Autodesk Inventor part; units mm, degrees
(part 3 of 3)
chamfer "面取り1" distance 0.1 angle 45 1544 edges at (166.6875, 1.524, 45.7073) (173.6108, 1.524, 45.7817) (173.6852, 1.524, 52.705) (173.6108, 1.524, 59.6283) (166.6875, 1.524, 59.7027) (159.7642, 1.524, 59.6283) (159.6898, 1.524, 52.705) (159.7642, 1.524, 45.7817) (166.6875, 0, 45.7073) (173.6108, 0, 45.7817) (173.6852, 0, 52.705) (173.6108, 0, 59.6283) (166.6875, 0, 59.7027) (159.7642, 0, 59.6283) (159.6898, 0, 52.705) (159.7642, 0, 45.7817) (147.6375, 1.524, 45.7073) (154.5608, 1.524, 45.7817) (154.6352, 1.524, 52.705) (154.5608, 1.524, 59.6283) (147.6375, 1.524, 59.7027) (140.7142, 1.524, 59.6283) (140.6398, 1.524, 52.705) (140.7142, 1.524, 45.7817) (147.6375, 0, 45.7073) (154.5608, 0, 45.7817) (154.6352, 0, 52.705) (154.5608, 0, 59.6283) (147.6375, 0, 59.7027) (140.7142, 0, 59.6283) (140.6398, 0, 52.705) (140.7142, 0, 45.7817) (128.5875, 0, 45.7073) (135.5108, 0, 45.7817) (135.5852, 0, 52.705) (135.5108, 0, 59.6283) (128.5875, 0, 59.7027) (121.6642, 0, 59.6283) (121.5898, 0, 52.705) (121.6642, 0, 45.7817) (128.5875, 1.524, 45.7073) (135.5108, 1.524, 45.7817) (135.5852, 1.524, 52.705) (135.5108, 1.524, 59.6283) (128.5875, 1.524, 59.7027) (121.6642, 1.524, 59.6283) (121.5898, 1.524, 52.705) (121.6642, 1.524, 45.7817) (147.6375, 1.524, 26.6573) (154.5608, 1.524, 26.7317) (154.6352, 1.524, 33.655) (154.5608, 1.524, 40.5783) (147.6375, 1.524, 40.6527) (140.7142, 1.524, 40.5783) (140.6398, 1.524, 33.655) (140.7142, 1.524, 26.7317) (147.6375, 0, 26.6573) (154.5608, 0, 26.7317) (154.6352, 0, 33.655) (154.5608, 0, 40.5783) (147.6375, 0, 40.6527) (140.7142, 0, 40.5783) (140.6398, 0, 33.655) (140.7142, 0, 26.7317) (97.63, 1.524, 45.7073) (104.5533, 1.524, 45.7817) (104.6277, 1.524, 52.705) (104.5533, 1.524, 59.6283) (97.63, 1.524, 59.7027) (90.7067, 1.524, 59.6283) (90.6323, 1.524, 52.705) (90.7067, 1.524, 45.7817) (97.63, 0, 45.7073) (104.5533, 0, 45.7817) (104.6277, 0, 52.705) (104.5533, 0, 59.6283) (97.63, 0, 59.7027) (90.7067, 0, 59.6283) (90.6323, 0, 52.705) (90.7067, 0, 45.7817) (73.8175, 1.524, 45.7073) (80.7408, 1.524, 45.7817) (80.8152, 1.524, 52.705) (80.7408, 1.524, 59.6283) (73.8175, 1.524, 59.7027) (66.8942, 1.524, 59.6283) (66.8198, 1.524, 52.705) (66.8942, 1.524, 45.7817) (73.8175, 0, 45.7073) (80.7408, 0, 45.7817) (80.8152, 0, 52.705) (80.7408, 0, 59.6283) (73.8175, 0, 59.7027) (66.8942, 0, 59.6283) (66.8198, 0, 52.705) (66.8942, 0, 45.7817) (78.4531, 0, 28.2829) (81.8787, 0, 28.3573) (81.9531, 0, 33.9979) (81.8787, 0, 39.6385) (78.4531, 0, 39.7129) (75.0275, 0, 39.6385) (74.9531, 0, 33.9979) (75.0275, 0, 28.3573) (78.4531, 1.524, 28.2829) (81.8787, 1.524, 28.3573) (81.9531, 1.524, 33.9979) (81.8787, 1.524, 39.6385) (78.4531, 1.524, 39.7129) (75.0275, 1.524, 39.6385) (74.9531, 1.524, 33.9979) (75.0275, 1.524, 28.3573) (90.4875, 1.524, 26.6573) (97.4108, 1.524, 26.7317) (97.4852, 1.524, 33.655) (97.4108, 1.524, 40.5783) (90.4875, 1.524, 40.6527) (83.5642, 1.524, 40.5783) (83.4898, 1.524, 33.655) (83.5642, 1.524, 26.7317) (90.4875, 0, 26.6573) (97.4108, 0, 26.7317) (97.4852, 0, 33.655) (97.4108, 0, 40.5783) (90.4875, 0, 40.6527) (83.5642, 0, 40.5783) (83.4898, 0, 33.655) (83.5642, 0, 26.7317) (102.5219, 0, 28.2829) (105.9475, 0, 28.3573) (106.0219, 0, 33.9979) (105.9475, 0, 39.6385) (102.5219, 0, 39.7129) (99.0963, 0, 39.6385) (99.0219, 0, 33.9979) (99.0963, 0, 28.3573) (102.5219, 1.524, 28.2829) (105.9475, 1.524, 28.3573) (106.0219, 1.524, 33.9979) (105.9475, 1.524, 39.6385) (102.5219, 1.524, 39.7129) (99.0963, 1.524, 39.6385) (99.0219, 1.524, 33.9979) (99.0963, 1.524, 28.3573) (97.9729, 0, 13.6144) (103.6135, 0, 13.6888) (103.6879, 0, 17.018) (103.6135, 0, 20.3472) (97.9729, 0, 20.4216) (92.3323, 0, 20.3472) (92.2579, 0, 17.018) (92.3323, 0, 13.6888) (97.9729, 1.524, 13.6144) (103.6135, 1.524, 13.6888) (103.6879, 1.524, 17.018) (103.6135, 1.524, 20.3472) (97.9729, 1.524, 20.4216) (92.3323, 1.524, 20.3472) (92.2579, 1.524, 17.018) (92.3323, 1.524, 13.6888) (97.63, 0, -1.9177) (104.5533, 0, -1.8433) (104.6277, 0, 5.08) (104.5533, 0, 12.0033) (97.63, 0, 12.0777) (90.7067, 0, 12.0033) (90.6323, 0, 5.08) (90.7067, 0, -1.8433) (97.63, 1.524, -1.9177) (104.5533, 1.524, -1.8433) (104.6277, 1.524, 5.08) (104.5533, 1.524, 12.0033) (97.63, 1.524, 12.0777) (90.7067, 1.524, 12.0033) (90.6323, 1.524, 5.08) (90.7067, 1.524, -1.8433) (97.9729, 0, -10.2616) (103.6135, 0, -10.1872) (103.6879, 0, -6.858) (103.6135, 0, -3.5288) (97.9729, 0, -3.4544) (92.3323, 0, -3.5288) (92.2579, 0, -6.858) (92.3323, 0, -10.1872) (97.9729, 1.524, -10.2616) (103.6135, 1.524, -10.1872) (103.6879, 1.524, -6.858) (103.6135, 1.524, -3.5288) (97.9729, 1.524, -3.4544) (92.3323, 1.524, -3.5288) (92.2579, 1.524, -6.858) (92.3323, 1.524, -10.1872) (100.0125, 0, -30.4927) (106.9358, 0, -30.4183) (107.0102, 0, -23.495) (106.9358, 0, -16.5717) (100.0125, 0, -16.4973) (93.0892, 0, -16.5717) (93.0148, 0, -23.495) (93.0892, 0, -30.4183) (100.0125, 1.524, -30.4927) (106.9358, 1.524, -30.4183) (107.0102, 1.524, -23.495) (106.9358, 1.524, -16.5717) (100.0125, 1.524, -16.4973) (93.0892, 1.524, -16.5717) (93.0148, 1.524, -23.495) (93.0892, 1.524, -30.4183) (100.0125, 0, -59.0677) (106.9358, 0, -58.9933) (107.0102, 0, -52.07) (106.9358, 0, -45.1467) (100.0125, 0, -45.0723) (93.0892, 0, -45.1467) (93.0148, 0, -52.07) (93.0892, 0, -58.9933) (100.0125, 1.524, -59.0677) (106.9358, 1.524, -58.9933) (107.0102, 1.524, -52.07) (106.9358, 1.524, -45.1467) (100.0125, 1.524, -45.0723) (93.0892, 1.524, -45.1467) (93.0148, 1.524, -52.07) (93.0892, 1.524, -58.9933) (128.5875, 0, -30.4927) (135.5108, 0, -30.4183) (135.5852, 0, -23.495) (135.5108, 0, -16.5717) (128.5875, 0, -16.4973) (121.6642, 0, -16.5717) (121.5898, 0, -23.495) (121.6642, 0, -30.4183) (128.5875, 1.524, -30.4927) (135.5108, 1.524, -30.4183) (135.5852, 1.524, -23.495) (135.5108, 1.524, -16.5717) (128.5875, 1.524, -16.4973) (121.6642, 1.524, -16.5717) (121.5898, 1.524, -23.495) (121.6642, 1.524, -30.4183) (128.5875, 0, -11.4427) (135.5108, 0, -11.3683) (135.5852, 0, -4.445) (135.5108, 0, 2.4783) (128.5875, 0, 2.5527) (121.6642, 0, 2.4783) (121.5898, 0, -4.445) (121.6642, 0, -11.3683) (128.5875, 1.524, -11.4427) (135.5108, 1.524, -11.3683) (135.5852, 1.524, -4.445) (135.5108, 1.524, 2.4783) (128.5875, 1.524, 2.5527) (121.6642, 1.524, 2.4783) (121.5898, 1.524, -4.445) (121.6642, 1.524, -11.3683) (147.6375, 1.524, -11.4427) (154.5608, 1.524, -11.3683) (154.6352, 1.524, -4.445) (154.5608, 1.524, 2.4783) (147.6375, 1.524, 2.5527) (140.7142, 1.524, 2.4783) (140.6398, 1.524, -4.445) (140.7142, 1.524, -11.3683) (147.6375, 0, -11.4427) (154.5608, 0, -11.3683) (154.6352, 0, -4.445) (154.5608, 0, 2.4783) (147.6375, 0, 2.5527) (140.7142, 0, 2.4783) (140.6398, 0, -4.445) (140.7142, 0, -11.3683) (147.6375, 0, -30.4927) (154.5608, 0, -30.4183) (154.6352, 0, -23.495) (154.5608, 0, -16.5717) (147.6375, 0, -16.4973) (140.7142, 0, -16.5717) (140.6398, 0, -23.495) (140.7142, 0, -30.4183) (147.6375, 1.524, -30.4927) (154.5608, 1.524, -30.4183) (154.6352, 1.524, -23.495) (154.5608, 1.524, -16.5717) (147.6375, 1.524, -16.4973) (140.7142, 1.524, -16.5717) (140.6398, 1.524, -23.495) (140.7142, 1.524, -30.4183) (166.6875, 0, -11.4427) (173.6108, 0, -11.3683) (173.6852, 0, -4.445) (173.6108, 0, 2.4783) (166.6875, 0, 2.5527) (159.7642, 0, 2.4783) (159.6898, 0, -4.445) (159.7642, 0, -11.3683) (166.6875, 1.524, -11.4427) (173.6108, 1.524, -11.3683) (173.6852, 1.524, -4.445) (173.6108, 1.524, 2.4783) (166.6875, 1.524, 2.5527) (159.7642, 1.524, 2.4783) (159.6898, 1.524, -4.445) (159.7642, 1.524, -11.3683) (166.6875, 0, -30.4927) (173.6108, 0, -30.4183) (173.6852, 0, -23.495) (173.6108, 0, -16.5717) (166.6875, 0, -16.4973) (159.7642, 0, -16.5717) (159.6898, 0, -23.495) (159.7642, 0, -30.4183) (166.6875, 1.524, -30.4927) (173.6108, 1.524, -30.4183) (173.6852, 1.524, -23.495) (173.6108, 1.524, -16.5717) (166.6875, 1.524, -16.4973) (159.7642, 1.524, -16.5717) (159.6898, 1.524, -23.495) (159.7642, 1.524, -30.4183) (80.9625, 0, -59.0677) (87.8858, 0, -58.9933) (87.9602, 0, -52.07) (87.8858, 0, -45.1467) (80.9625, 0, -45.0723) (74.0392, 0, -45.1467) (73.9648, 0, -52.07) (74.0392, 0, -58.9933) (80.9625, 1.524, -59.0677) (87.8858, 1.524, -58.9933) (87.9602, 1.524, -52.07) (87.8858, 1.524, -45.1467) (80.9625, 1.524, -45.0723) (74.0392, 1.524, -45.1467) (73.9648, 1.524, -52.07) (74.0392, 1.524, -58.9933) (80.9625, 1.524, -30.4927) (87.8858, 1.524, -30.4183) (87.9602, 1.524, -23.495) (87.8858, 1.524, -16.5717) (80.9625, 1.524, -16.4973) (74.0392, 1.524, -16.5717) (73.9648, 1.524, -23.495) (74.0392, 1.524, -30.4183) (80.9625, 0, -30.4927) (87.8858, 0, -30.4183) (87.9602, 0, -23.495) (87.8858, 0, -16.5717) (80.9625, 0, -16.4973) (74.0392, 0, -16.5717) (73.9648, 0, -23.495) (74.0392, 0, -30.4183) (71.4375, 0, -11.4427) (78.3608, 0, -11.3683) (78.4352, 0, -4.445) (78.3608, 0, 2.4783) (71.4375, 0, 2.5527) (64.5142, 0, 2.4783) (64.4398, 0, -4.445) (64.5142, 0, -11.3683) (71.4375, 1.524, -11.4427) (78.3608, 1.524, -11.3683) (78.4352, 1.524, -4.445) (78.3608, 1.524, 2.4783) (71.4375, 1.524, 2.5527) (64.5142, 1.524, 2.4783) (64.4398, 1.524, -4.445) (64.5142, 1.524, -11.3683) (76.2, 0, 7.6073) (83.1233, 0, 7.6817) (83.1977, 0, 14.605) (83.1233, 0, 21.5283) (76.2, 0, 21.6027) (69.2767, 0, 21.5283) (69.2023, 0, 14.605) (69.2767, 0, 7.6817) (76.2, 1.524, 7.6073) (83.1233, 1.524, 7.6817) (83.1977, 1.524, 14.605) (83.1233, 1.524, 21.5283) (76.2, 1.524, 21.6027) (69.2767, 1.524, 21.5283) (69.2023, 1.524, 14.605) (69.2767, 1.524, 7.6817) (50.005, 0, 45.7073) (56.9283, 0, 45.7817) (57.0027, 0, 52.705) (56.9283, 0, 59.6283) (50.005, 0, 59.7027) (43.0817, 0, 59.6283) (43.0073, 0, 52.705) (43.0817, 0, 45.7817) (50.005, 1.524, 45.7073) (56.9283, 1.524, 45.7817) (57.0027, 1.524, 52.705) (56.9283, 1.524, 59.6283) (50.005, 1.524, 59.7027) (43.0817, 1.524, 59.6283) (43.0073, 1.524, 52.705) (43.0817, 1.524, 45.7817) (61.9125, 0, 26.6573) (68.8358, 0, 26.7317) (68.9102, 0, 33.655) (68.8358, 0, 40.5783) (61.9125, 0, 40.6527) (54.9892, 0, 40.5783) (54.9148, 0, 33.655) (54.9892, 0, 26.7317) (61.9125, 1.524, 26.6573) (68.8358, 1.524, 26.7317) (68.9102, 1.524, 33.655) (68.8358, 1.524, 40.5783) (61.9125, 1.524, 40.6527) (54.9892, 1.524, 40.5783) (54.9148, 1.524, 33.655) (54.9892, 1.524, 26.7317) (57.15, 0, 7.6073) (64.0733, 0, 7.6817) (64.1477, 0, 14.605) (64.0733, 0, 21.5283) (57.15, 0, 21.6027) (50.2267, 0, 21.5283) (50.1523, 0, 14.605) (50.2267, 0, 7.6817) (57.15, 1.524, 7.6073) (64.0733, 1.524, 7.6817) (64.1477, 1.524, 14.605) (64.0733, 1.524, 21.5283) (57.15, 1.524, 21.6027) (50.2267, 1.524, 21.5283) (50.1523, 1.524, 14.605) (50.2267, 1.524, 7.6817) (52.3875, 0, -11.4427) (59.3108, 0, -11.3683) (59.3852, 0, -4.445) (59.3108, 0, 2.4783) (52.3875, 0, 2.5527) (45.4642, 0, 2.4783) (45.3898, 0, -4.445) (45.4642, 0, -11.3683) (52.3875, 1.524, -11.4427) (59.3108, 1.524, -11.3683) (59.3852, 1.524, -4.445) (59.3108, 1.524, 2.4783) (52.3875, 1.524, 2.5527) (45.4642, 1.524, 2.4783) (45.3898, 1.524, -4.445) (45.4642, 1.524, -11.3683) (61.9125, 0, -30.4927) (68.8358, 0, -30.4183) (68.9102, 0, -23.495) (68.8358, 0, -16.5717) (61.9125, 0, -16.4973) (54.9892, 0, -16.5717) (54.9148, 0, -23.495) (54.9892, 0, -30.4183) (61.9125, 1.524, -30.4927) (68.8358, 1.524, -30.4183) (68.9102, 1.524, -23.495) (68.8358, 1.524, -16.5717) (61.9125, 1.524, -16.4973) (54.9892, 1.524, -16.5717) (54.9148, 1.524, -23.495) (54.9892, 1.524, -30.4183) (61.9125, 0, -59.0677) (68.8358, 0, -58.9933) (68.9102, 0, -52.07) (68.8358, 0, -45.1467) (61.9125, 0, -45.0723) (54.9892, 0, -45.1467) (54.9148, 0, -52.07) (54.9892, 0, -58.9933) (61.9125, 1.524, -59.0677) (68.8358, 1.524, -58.9933) (68.9102, 1.524, -52.07) (68.8358, 1.524, -45.1467) (61.9125, 1.524, -45.0723) (54.9892, 1.524, -45.1467) (54.9148, 1.524, -52.07) (54.9892, 1.524, -58.9933) (42.8625, 1.524, -59.0677) (49.7858, 1.524, -58.9933) (49.8602, 1.524, -52.07) (49.7858, 1.524, -45.1467) (42.8625, 1.524, -45.0723) (35.9392, 1.524, -45.1467) (35.8648, 1.524, -52.07) (35.9392, 1.524, -58.9933) (42.8625, 0, -59.0677) (49.7858, 0, -58.9933) (49.8602, 0, -52.07) (49.7858, 0, -45.1467) (42.8625, 0, -45.0723) (35.9392, 0, -45.1467) (35.8648, 0, -52.07) (35.9392, 0, -58.9933) (42.8625, 0, -30.4927) (49.7858, 0, -30.4183) (49.8602, 0, -23.495) (49.7858, 0, -16.5717) (42.8625, 0, -16.4973) (35.9392, 0, -16.5717) (35.8648, 0, -23.495) (35.9392, 0, -30.4183) (42.8625, 1.524, -30.4927) (49.7858, 1.524, -30.4183) (49.8602, 1.524, -23.495) (49.7858, 1.524, -16.5717) (42.8625, 1.524, -16.4973) (35.9392, 1.524, -16.5717) (35.8648, 1.524, -23.495) (35.9392, 1.524, -30.4183) (42.8625, 0, 26.6573) (49.7858, 0, 26.7317) (49.8602, 0, 33.655) (49.7858, 0, 40.5783) (42.8625, 0, 40.6527) (35.9392, 0, 40.5783) (35.8648, 0, 33.655) (35.9392, 0, 26.7317) (42.8625, 1.524, 26.6573) (49.7858, 1.524, 26.7317) (49.8602, 1.524, 33.655) (49.7858, 1.524, 40.5783) (42.8625, 1.524, 40.6527) (35.9392, 1.524, 40.5783) (35.8648, 1.524, 33.655) (35.9392, 1.524, 26.7317) (38.1, 0, 7.6073) (45.0233, 0, 7.6817) (45.0977, 0, 14.605) (45.0233, 0, 21.5283) (38.1, 0, 21.6027) (31.1767, 0, 21.5283) (31.1023, 0, 14.605) (31.1767, 0, 7.6817) (38.1, 1.524, 7.6073) (45.0233, 1.524, 7.6817) (45.0977, 1.524, 14.605) (45.0233, 1.524, 21.5283) (38.1, 1.524, 21.6027) (31.1767, 1.524, 21.5283) (31.1023, 1.524, 14.605) (31.1767, 1.524, 7.6817) (33.3375, 0, -11.4427) (40.2608, 0, -11.3683) (40.3352, 0, -4.445) (40.2608, 0, 2.4783) (33.3375, 0, 2.5527) (26.4142, 0, 2.4783) (26.3398, 0, -4.445) (26.4142, 0, -11.3683) (33.3375, 1.524, -11.4427) (40.2608, 1.524, -11.3683) (40.3352, 1.524, -4.445) (40.2608, 1.524, 2.4783) (33.3375, 1.524, 2.5527) (26.4142, 1.524, 2.4783) (26.3398, 1.524, -4.445) (26.4142, 1.524, -11.3683) (23.8125, 0, -30.4927) (30.7358, 0, -30.4183) (30.8102, 0, -23.495) (30.7358, 0, -16.5717) (23.8125, 0, -16.4973) (16.8892, 0, -16.5717) (16.8148, 0, -23.495) (16.8892, 0, -30.4183) (23.8125, 1.524, -30.4927) (30.7358, 1.524, -30.4183) (30.8102, 1.524, -23.495) (30.7358, 1.524, -16.5717) (23.8125, 1.524, -16.4973) (16.8892, 1.524, -16.5717) (16.8148, 1.524, -23.495) (16.8892, 1.524, -30.4183) (26.1925, 0, 45.7073) (33.1158, 0, 45.7817) (33.1902, 0, 52.705) (33.1158, 0, 59.6283) (26.1925, 0, 59.7027) (19.2692, 0, 59.6283) (19.1948, 0, 52.705) (19.2692, 0, 45.7817) (26.1925, 1.524, 45.7073) (33.1158, 1.524, 45.7817) (33.1902, 1.524, 52.705) (33.1158, 1.524, 59.6283) (26.1925, 1.524, 59.7027) (19.2692, 1.524, 59.6283) (19.1948, 1.524, 52.705) (19.2692, 1.524, 45.7817) (23.8125, 0, 26.6573) (30.7358, 0, 26.7317) (30.8102, 0, 33.655) (30.7358, 0, 40.5783) (23.8125, 0, 40.6527) (16.8892, 0, 40.5783) (16.8148, 0, 33.655) (16.8892, 0, 26.7317) (23.8125, 1.524, 26.6573) (30.7358, 1.524, 26.7317) (30.8102, 1.524, 33.655) (30.7358, 1.524, 40.5783) (23.8125, 1.524, 40.6527) (16.8892, 1.524, 40.5783) (16.8148, 1.524, 33.655) (16.8892, 1.524, 26.7317) (19.05, 0, 7.6073) (25.9733, 0, 7.6817) (26.0477, 0, 14.605) (25.9733, 0, 21.5283) (19.05, 0, 21.6027) (12.1267, 0, 21.5283) (12.0523, 0, 14.605) (12.1267, 0, 7.6817) (19.05, 1.524, 7.6073) (25.9733, 1.524, 7.6817) (26.0477, 1.524, 14.605) (25.9733, 1.524, 21.5283) (19.05, 1.524, 21.6027) (12.1267, 1.524, 21.5283) (12.0523, 1.524, 14.605) (12.1267, 1.524, 7.6817) (14.2875, 0, -11.4427) (21.2108, 0, -11.3683) (21.2852, 0, -4.445) (21.2108, 0, 2.4783) (14.2875, 0, 2.5527) (7.3642, 0, 2.4783) (7.2898, 0, -4.445) (7.3642, 0, -11.3683) (14.2875, 1.524, -11.4427) (21.2108, 1.524, -11.3683) (21.2852, 1.524, -4.445) (21.2108, 1.524, 2.4783) (14.2875, 1.524, 2.5527) (7.3642, 1.524, 2.4783) (7.2898, 1.524, -4.445) (7.3642, 1.524, -11.3683) (14.2875, 0, -59.0677) (21.2108, 0, -58.9933) (21.2852, 0, -52.07) (21.2108, 0, -45.1467) (14.2875, 0, -45.0723) (7.3642, 0, -45.1467) (7.2898, 0, -52.07) (7.3642, 0, -58.9933) (14.2875, 1.524, -59.0677) (21.2108, 1.524, -58.9933) (21.2852, 1.524, -52.07) (21.2108, 1.524, -45.1467) (14.2875, 1.524, -45.0723) (7.3642, 1.524, -45.1467) (7.2898, 1.524, -52.07) (7.3642, 1.524, -58.9933) (4.7625, 0, -30.4927) (11.6858, 0, -30.4183) (11.7602, 0, -23.495) (11.6858, 0, -16.5717) (4.7625, 0, -16.4973) (-2.1608, 0, -16.5717) (-2.2352, 0, -23.495) (-2.1608, 0, -30.4183) (4.7625, 1.524, -30.4927) (11.6858, 1.524, -30.4183) (11.7602, 1.524, -23.495) (11.6858, 1.524, -16.5717) (4.7625, 1.524, -16.4973) (-2.1608, 1.524, -16.5717) (-2.2352, 1.524, -23.495) (-2.1608, 1.524, -30.4183) (-4.7625, 0, -59.0677) (2.1608, 0, -58.9933) (2.2352, 0, -52.07) (2.1608, 0, -45.1467) (-4.7625, 0, -45.0723) (-11.6858, 0, -45.1467) (-11.7602, 0, -52.07) (-11.6858, 0, -58.9933) (-4.7625, 1.524, -59.0677) (2.1608, 1.524, -58.9933) (2.2352, 1.524, -52.07) (2.1608, 1.524, -45.1467) (-4.7625, 1.524, -45.0723) (-11.6858, 1.524, -45.1467) (-11.7602, 1.524, -52.07) (-11.6858, 1.524, -58.9933) (4.7625, 0, 26.6573) (11.6858, 0, 26.7317) (11.7602, 0, 33.655) (11.6858, 0, 40.5783) (4.7625, 0, 40.6527) (-2.1608, 0, 40.5783) (-2.2352, 0, 33.655) (-2.1608, 0, 26.7317) (4.7625, 1.524, 26.6573) (11.6858, 1.524, 26.7317) (11.7602, 1.524, 33.655) (11.6858, 1.524, 40.5783) (4.7625, 1.524, 40.6527) (-2.1608, 1.524, 40.5783) (-2.2352, 1.524, 33.655) (-2.1608, 1.524, 26.7317) (0, 0, 7.6073) (6.9233, 0, 7.6817) (6.9977, 0, 14.605) (6.9233, 0, 21.5283) (0, 0, 21.6027) (-6.9233, 0, 21.5283) (-6.9977, 0, 14.605) (-6.9233, 0, 7.6817) (0, 1.524, 7.6073) (6.9233, 1.524, 7.6817) (6.9977, 1.524, 14.605) (6.9233, 1.524, 21.5283) (0, 1.524, 21.6027) (-6.9233, 1.524, 21.5283) (-6.9977, 1.524, 14.605) (-6.9233, 1.524, 7.6817) (-4.7625, 0, -11.4427) (2.1608, 0, -11.3683) (2.2352, 0, -4.445) (2.1608, 0, 2.4783) (-4.7625, 0, 2.5527) (-11.6858, 0, 2.4783) (-11.7602, 0, -4.445) (-11.6858, 0, -11.3683) (-4.7625, 1.524, -11.4427) (2.1608, 1.524, -11.3683) (2.2352, 1.524, -4.445) (2.1608, 1.524, 2.4783) (-4.7625, 1.524, 2.5527) (-11.6858, 1.524, 2.4783) (-11.7602, 1.524, -4.445) (-11.6858, 1.524, -11.3683) (-14.2875, 0, -30.4927) (-7.3642, 0, -30.4183) (-7.2898, 0, -23.495) (-7.3642, 0, -16.5717) (-14.2875, 0, -16.4973) (-21.2108, 0, -16.5717) (-21.2852, 0, -23.495) (-21.2108, 0, -30.4183) (-14.2875, 1.524, -30.4927) (-7.3642, 1.524, -30.4183) (-7.2898, 1.524, -23.495) (-7.3642, 1.524, -16.5717) (-14.2875, 1.524, -16.4973) (-21.2108, 1.524, -16.5717) (-21.2852, 1.524, -23.495) (-21.2108, 1.524, -30.4183) (-7.9375, 0, 47.3329) (-4.5119, 0, 47.4073) (-4.4375, 0, 53.0479) (-4.5119, 0, 58.6885) (-7.9375, 0, 58.7629) (-11.3631, 0, 58.6885) (-11.4375, 0, 53.0479) (-11.3631, 0, 47.4073) (-7.9375, 1.524, 47.3329) (-4.5119, 1.524, 47.4073) (-4.4375, 1.524, 53.0479) (-4.5119, 1.524, 58.6885) (-7.9375, 1.524, 58.7629) (-11.3631, 1.524, 58.6885) (-11.4375, 1.524, 53.0479) (-11.3631, 1.524, 47.4073) (-14.2875, 0, 26.6573) (-7.3642, 0, 26.7317) (-7.2898, 0, 33.655) (-7.3642, 0, 40.5783) (-14.2875, 0, 40.6527) (-21.2108, 0, 40.5783) (-21.2852, 0, 33.655) (-21.2108, 0, 26.7317) (-14.2875, 1.524, 26.6573) (-7.3642, 1.524, 26.7317) (-7.2898, 1.524, 33.655) (-7.3642, 1.524, 40.5783) (-14.2875, 1.524, 40.6527) (-21.2108, 1.524, 40.5783) (-21.2852, 1.524, 33.655) (-21.2108, 1.524, 26.7317) (-19.05, 0, 7.6073) (-12.1267, 0, 7.6817) (-12.0523, 0, 14.605) (-12.1267, 0, 21.5283) (-19.05, 0, 21.6027) (-25.9733, 0, 21.5283) (-26.0477, 0, 14.605) (-25.9733, 0, 7.6817) (-19.05, 1.524, 7.6073) (-12.1267, 1.524, 7.6817) (-12.0523, 1.524, 14.605) (-12.1267, 1.524, 21.5283) (-19.05, 1.524, 21.6027) (-25.9733, 1.524, 21.5283) (-26.0477, 1.524, 14.605) (-25.9733, 1.524, 7.6817) (-23.8125, 0, -11.4427) (-16.8892, 0, -11.3683) (-16.8148, 0, -4.445) (-16.8892, 0, 2.4783) (-23.8125, 0, 2.5527) (-30.7358, 0, 2.4783) (-30.8102, 0, -4.445) (-30.7358, 0, -11.3683) (-23.8125, 1.524, -11.4427) (-16.8892, 1.524, -11.3683) (-16.8148, 1.524, -4.445) (-16.8892, 1.524, 2.4783) (-23.8125, 1.524, 2.5527) (-30.7358, 1.524, 2.4783) (-30.8102, 1.524, -4.445) (-30.7358, 1.524, -11.3683) (-23.8125, 0, -59.0677) (-16.8892, 0, -58.9933) (-16.8148, 0, -52.07) (-16.8892, 0, -45.1467) (-23.8125, 0, -45.0723) (-30.7358, 0, -45.1467) (-30.8102, 0, -52.07) (-30.7358, 0, -58.9933) (-23.8125, 1.524, -59.0677) (-16.8892, 1.524, -58.9933) (-16.8148, 1.524, -52.07) (-16.8892, 1.524, -45.1467) (-23.8125, 1.524, -45.0723) (-30.7358, 1.524, -45.1467) (-30.8102, 1.524, -52.07) (-30.7358, 1.524, -58.9933) (-21.3031, 0, 47.3329) (-17.8775, 0, 47.4073) (-17.8031, 0, 53.0479) (-17.8775, 0, 58.6885) (-21.3031, 0, 58.7629) (-24.7287, 0, 58.6885) (-24.8031, 0, 53.0479) (-24.7287, 0, 47.4073) (-21.3031, 1.524, 47.3329) (-17.8775, 1.524, 47.4073) (-17.8031, 1.524, 53.0479) (-17.8775, 1.524, 58.6885) (-21.3031, 1.524, 58.7629) (-24.7287, 1.524, 58.6885) (-24.8031, 1.524, 53.0479) (-24.7287, 1.524, 47.4073) (-33.3375, 0, -30.4927) (-26.4142, 0, -30.4183) (-26.3398, 0, -23.495) (-26.4142, 0, -16.5717) (-33.3375, 0, -16.4973) (-40.2608, 0, -16.5717) (-40.3352, 0, -23.495) (-40.2608, 0, -30.4183) (-33.3375, 1.524, -30.4927) (-26.4142, 1.524, -30.4183) (-26.3398, 1.524, -23.495) (-26.4142, 1.524, -16.5717) (-33.3375, 1.524, -16.4973) (-40.2608, 1.524, -16.5717) (-40.3352, 1.524, -23.495) (-40.2608, 1.524, -30.4183) (-42.8625, 0, -59.0677) (-35.9392, 0, -58.9933) (-35.8648, 0, -52.07) (-35.9392, 0, -45.1467) (-42.8625, 0, -45.0723) (-49.7858, 0, -45.1467) (-49.8602, 0, -52.07) (-49.7858, 0, -58.9933) (-42.8625, 1.524, -59.0677) (-35.9392, 1.524, -58.9933) (-35.8648, 1.524, -52.07) (-35.9392, 1.524, -45.1467) (-42.8625, 1.524, -45.0723) (-49.7858, 1.524, -45.1467) (-49.8602, 1.524, -52.07) (-49.7858, 1.524, -58.9933) (-33.3375, 0, 45.7073) (-26.4142, 0, 45.7817) (-26.3398, 0, 52.705) (-26.4142, 0, 59.6283) (-33.3375, 0, 59.7027) (-40.2608, 0, 59.6283) (-40.3352, 0, 52.705) (-40.2608, 0, 45.7817) (-33.3375, 1.524, 45.7073) (-26.4142, 1.524, 45.7817) (-26.3398, 1.524, 52.705) (-26.4142, 1.524, 59.6283) (-33.3375, 1.524, 59.7027) (-40.2608, 1.524, 59.6283) (-40.3352, 1.524, 52.705) (-40.2608, 1.524, 45.7817) (-33.3375, 0, 26.6573) (-26.4142, 0, 26.7317) (-26.3398, 0, 33.655) (-26.4142, 0, 40.5783) (-33.3375, 0, 40.6527) (-40.2608, 0, 40.5783) (-40.3352, 0, 33.655) (-40.2608, 0, 26.7317) (-52.3875, 1.524, -30.4927) (-45.4642, 1.524, -30.4183) (-45.3898, 1.524, -23.495) (-45.4642, 1.524, -16.5717) (-52.3875, 1.524, -16.4973) (-59.3108, 1.524, -16.5717) (-59.3852, 1.524, -23.495) (-59.3108, 1.524, -30.4183) (-52.3875, 0, -30.4927) (-45.4642, 0, -30.4183) (-45.3898, 0, -23.495) (-45.4642, 0, -16.5717) (-52.3875, 0, -16.4973) (-59.3108, 0, -16.5717) (-59.3852, 0, -23.495) (-59.3108, 0, -30.4183) (-42.8625, 1.524, -11.4427) (-35.9392, 1.524, -11.3683) (-35.8648, 1.524, -4.445) (-35.9392, 1.524, 2.4783) (-42.8625, 1.524, 2.5527) (-49.7858, 1.524, 2.4783) (-49.8602, 1.524, -4.445) (-49.7858, 1.524, -11.3683) (-42.8625, 0, -11.4427) (-35.9392, 0, -11.3683) (-35.8648, 0, -4.445) (-35.9392, 0, 2.4783) (-42.8625, 0, 2.5527) (-49.7858, 0, 2.4783) (-49.8602, 0, -4.445) (-49.7858, 0, -11.3683) (-38.1, 1.524, 7.6073) (-31.1767, 1.524, 7.6817) (-31.1023, 1.524, 14.605) (-31.1767, 1.524, 21.5283) (-38.1, 1.524, 21.6027) (-45.0233, 1.524, 21.5283) (-45.0977, 1.524, 14.605) (-45.0233, 1.524, 7.6817) (-38.1, 0, 7.6073) (-31.1767, 0, 7.6817) (-31.1023, 0, 14.605) (-31.1767, 0, 21.5283) (-38.1, 0, 21.6027) (-45.0233, 0, 21.5283) (-45.0977, 0, 14.605) (-45.0233, 0, 7.6817) (-45.3719, 1.524, 47.3329) (-41.9463, 1.524, 47.4073) (-41.8719, 1.524, 53.0479) (-41.9463, 1.524, 58.6885) (-45.3719, 1.524, 58.7629) (-48.7975, 1.524, 58.6885) (-48.8719, 1.524, 53.0479) (-48.7975, 1.524, 47.4073) (-45.3719, 0, 47.3329) (-41.9463, 0, 47.4073) (-41.8719, 0, 53.0479) (-41.9463, 0, 58.6885) (-45.3719, 0, 58.7629) (-48.7975, 0, 58.6885) (-48.8719, 0, 53.0479) (-48.7975, 0, 47.4073) (-52.3875, 0, 26.6573) (-45.4642, 0, 26.7317) (-45.3898, 0, 33.655) (-45.4642, 0, 40.5783) (-52.3875, 0, 40.6527) (-59.3108, 0, 40.5783) (-59.3852, 0, 33.655) (-59.3108, 0, 26.7317) (-52.3875, 1.524, 26.6573) (-45.4642, 1.524, 26.7317) (-45.3898, 1.524, 33.655) (-45.4642, 1.524, 40.5783) (-52.3875, 1.524, 40.6527) (-59.3108, 1.524, 40.5783) (-59.3852, 1.524, 33.655) (-59.3108, 1.524, 26.7317) (-58.7375, 0, 47.3329) (-55.3119, 0, 47.4073) (-55.2375, 0, 53.0479) (-55.3119, 0, 58.6885) (-58.7375, 0, 58.7629) (-62.1631, 0, 58.6885) (-62.2375, 0, 53.0479) (-62.1631, 0, 47.4073) (-58.7375, 1.524, 47.3329) (-55.3119, 1.524, 47.4073) (-55.2375, 1.524, 53.0479) (-55.3119, 1.524, 58.6885) (-58.7375, 1.524, 58.7629) (-62.1631, 1.524, 58.6885) (-62.2375, 1.524, 53.0479) (-62.1631, 1.524, 47.4073) (-57.15, 0, 7.6073) (-50.2267, 0, 7.6817) (-50.1523, 0, 14.605) (-50.2267, 0, 21.5283) (-57.15, 0, 21.6027) (-64.0733, 0, 21.5283) (-64.1477, 0, 14.605) (-64.0733, 0, 7.6817) (-57.15, 1.524, 7.6073) (-50.2267, 1.524, 7.6817) (-50.1523, 1.524, 14.605) (-50.2267, 1.524, 21.5283) (-57.15, 1.524, 21.6027) (-64.0733, 1.524, 21.5283) (-64.1477, 1.524, 14.605) (-64.0733, 1.524, 7.6817) (-61.9125, 0, -11.4427) (-54.9892, 0, -11.3683) (-54.9148, 0, -4.445) (-54.9892, 0, 2.4783) (-61.9125, 0, 2.5527) (-68.8358, 0, 2.4783) (-68.9102, 0, -4.445) (-68.8358, 0, -11.3683) (-61.9125, 1.524, -11.4427) (-54.9892, 1.524, -11.3683) (-54.9148, 1.524, -4.445) (-54.9892, 1.524, 2.4783) (-61.9125, 1.524, 2.5527) (-68.8358, 1.524, 2.4783) (-68.9102, 1.524, -4.445) (-68.8358, 1.524, -11.3683) (-71.4375, 0, -59.0677) (-64.5142, 0, -58.9933) (-64.4398, 0, -52.07) (-64.5142, 0, -45.1467) (-71.4375, 0, -45.0723) (-78.3608, 0, -45.1467) (-78.4352, 0, -52.07) (-78.3608, 0, -58.9933) (-71.4375, 1.524, -59.0677) (-64.5142, 1.524, -58.9933) (-64.4398, 1.524, -52.07) (-64.5142, 1.524, -45.1467) (-71.4375, 1.524, -45.0723) (-78.3608, 1.524, -45.1467) (-78.4352, 1.524, -52.07) (-78.3608, 1.524, -58.9933) (-71.4375, 1.524, -30.4927) (-64.5142, 1.524, -30.4183) (-64.4398, 1.524, -23.495) (-64.5142, 1.524, -16.5717) (-71.4375, 1.524, -16.4973) (-78.3608, 1.524, -16.5717) (-78.4352, 1.524, -23.495) (-78.3608, 1.524, -30.4183) (-71.4375, 0, -30.4927) (-64.5142, 0, -30.4183) (-64.4398, 0, -23.495) (-64.5142, 0, -16.5717) (-71.4375, 0, -16.4973) (-78.3608, 0, -16.5717) (-78.4352, 0, -23.495) (-78.3608, 0, -30.4183) (-71.4375, 0, 26.6573) (-64.5142, 0, 26.7317) (-64.4398, 0, 33.655) (-64.5142, 0, 40.5783) (-71.4375, 0, 40.6527) (-78.3608, 0, 40.5783) (-78.4352, 0, 33.655) (-78.3608, 0, 26.7317) (-71.4375, 1.524, 26.6573) (-64.5142, 1.524, 26.7317) (-64.4398, 1.524, 33.655) (-64.5142, 1.524, 40.5783) (-71.4375, 1.524, 40.6527) (-78.3608, 1.524, 40.5783) (-78.4352, 1.524, 33.655) (-78.3608, 1.524, 26.7317) (-76.2, 0, 7.6073) (-69.2767, 0, 7.6817) (-69.2023, 0, 14.605) (-69.2767, 0, 21.5283) (-76.2, 0, 21.6027) (-83.1233, 0, 21.5283) (-83.1977, 0, 14.605) (-83.1233, 0, 7.6817) (-76.2, 1.524, 7.6073) (-69.2767, 1.524, 7.6817) (-69.2023, 1.524, 14.605) (-69.2767, 1.524, 21.5283) (-76.2, 1.524, 21.6027) (-83.1233, 1.524, 21.5283) (-83.1977, 1.524, 14.605) (-83.1233, 1.524, 7.6817) (-80.9625, 0, -11.4427) (-74.0392, 0, -11.3683) (-73.9648, 0, -4.445) (-74.0392, 0, 2.4783) (-80.9625, 0, 2.5527) (-87.8858, 0, 2.4783) (-87.9602, 0, -4.445) (-87.8858, 0, -11.3683) (-80.9625, 1.524, -11.4427) (-74.0392, 1.524, -11.3683) (-73.9648, 1.524, -4.445) (-74.0392, 1.524, 2.4783) (-80.9625, 1.524, 2.5527) (-87.8858, 1.524, 2.4783) (-87.9602, 1.524, -4.445) (-87.8858, 1.524, -11.3683) (-90.4875, 0, -59.0677) (-83.5642, 0, -58.9933) (-83.4898, 0, -52.07) (-83.5642, 0, -45.1467) (-90.4875, 0, -45.0723) (-97.4108, 0, -45.1467) (-97.4852, 0, -52.07) (-97.4108, 0, -58.9933) (-90.4875, 1.524, -59.0677) (-83.5642, 1.524, -58.9933) (-83.4898, 1.524, -52.07) (-83.5642, 1.524, -45.1467) (-90.4875, 1.524, -45.0723) (-97.4108, 1.524, -45.1467) (-97.4852, 1.524, -52.07) (-97.4108, 1.524, -58.9933) (-90.4875, 0, -30.4927) (-83.5642, 0, -30.4183) (-83.4898, 0, -23.495) (-83.5642, 0, -16.5717) (-90.4875, 0, -16.4973) (-97.4108, 0, -16.5717) (-97.4852, 0, -23.495) (-97.4108, 0, -30.4183) (-90.4875, 1.524, -30.4927) (-83.5642, 1.524, -30.4183) (-83.4898, 1.524, -23.495) (-83.5642, 1.524, -16.5717) (-90.4875, 1.524, -16.4973) (-97.4108, 1.524, -16.5717) (-97.4852, 1.524, -23.495) (-97.4108, 1.524, -30.4183) (-90.4875, 0, 26.6573) (-83.5642, 0, 26.7317) (-83.4898, 0, 33.655) (-83.5642, 0, 40.5783) (-90.4875, 0, 40.6527) (-97.4108, 0, 40.5783) (-97.4852, 0, 33.655) (-97.4108, 0, 26.7317) (-90.4875, 1.524, 26.6573) (-83.5642, 1.524, 26.7317) (-83.4898, 1.524, 33.655) (-83.5642, 1.524, 40.5783) (-90.4875, 1.524, 40.6527) (-97.4108, 1.524, 40.5783) (-97.4852, 1.524, 33.655) (-97.4108, 1.524, 26.7317) (-92.87, 1.524, 45.7073) (-85.9467, 1.524, 45.7817) (-85.8723, 1.524, 52.705) (-85.9467, 1.524, 59.6283) (-92.87, 1.524, 59.7027) (-99.7933, 1.524, 59.6283) (-99.8677, 1.524, 52.705) (-99.7933, 1.524, 45.7817) (-92.87, 0, 45.7073) (-85.9467, 0, 45.7817) (-85.8723, 0, 52.705) (-85.9467, 0, 59.6283) (-92.87, 0, 59.7027) (-99.7933, 0, 59.6283) (-99.8677, 0, 52.705) (-99.7933, 0, 45.7817) (-95.25, 0, 7.6073) (-88.3267, 0, 7.6817) (-88.2523, 0, 14.605) (-88.3267, 0, 21.5283) (-95.25, 0, 21.6027) (-102.1733, 0, 21.5283) (-102.2477, 0, 14.605) (-102.1733, 0, 7.6817) (-95.25, 1.524, 7.6073) (-88.3267, 1.524, 7.6817) (-88.2523, 1.524, 14.605) (-88.3267, 1.524, 21.5283) (-95.25, 1.524, 21.6027) (-102.1733, 1.524, 21.5283) (-102.2477, 1.524, 14.605) (-102.1733, 1.524, 7.6817) (-100.0125, 0, -11.4427) (-93.0892, 0, -11.3683) (-93.0148, 0, -4.445) (-93.0892, 0, 2.4783) (-100.0125, 0, 2.5527) (-106.9358, 0, 2.4783) (-107.0102, 0, -4.445) (-106.9358, 0, -11.3683) (-100.0125, 1.524, -11.4427) (-93.0892, 1.524, -11.3683) (-93.0148, 1.524, -4.445) (-93.0892, 1.524, 2.4783) (-100.0125, 1.524, 2.5527) (-106.9358, 1.524, 2.4783) (-107.0102, 1.524, -4.445) (-106.9358, 1.524, -11.3683) (-109.5375, 1.524, 26.6573) (-102.6142, 1.524, 26.7317) (-102.5398, 1.524, 33.655) (-102.6142, 1.524, 40.5783) (-109.5375, 1.524, 40.6527) (-116.4608, 1.524, 40.5783) (-116.5352, 1.524, 33.655) (-116.4608, 1.524, 26.7317) (-109.5375, 0, 26.6573) (-102.6142, 0, 26.7317) (-102.5398, 0, 33.655) (-102.6142, 0, 40.5783) (-109.5375, 0, 40.6527) (-116.4608, 0, 40.5783) (-116.5352, 0, 33.655) (-116.4608, 0, 26.7317) (-116.6825, 0, 45.7073) (-109.7592, 0, 45.7817) (-109.6848, 0, 52.705) (-109.7592, 0, 59.6283) (-116.6825, 0, 59.7027) (-123.6058, 0, 59.6283) (-123.6802, 0, 52.705) (-123.6058, 0, 45.7817) (-116.6825, 1.524, 45.7073) (-109.7592, 1.524, 45.7817) (-109.6848, 1.524, 52.705) (-109.7592, 1.524, 59.6283) (-116.6825, 1.524, 59.7027) (-123.6058, 1.524, 59.6283) (-123.6802, 1.524, 52.705) (-123.6058, 1.524, 45.7817) (-114.3, 0, 7.6073) (-107.3767, 0, 7.6817) (-107.3023, 0, 14.605) (-107.3767, 0, 21.5283) (-114.3, 0, 21.6027) (-121.2233, 0, 21.5283) (-121.2977, 0, 14.605) (-121.2233, 0, 7.6817) (-114.3, 1.524, 7.6073) (-107.3767, 1.524, 7.6817) (-107.3023, 1.524, 14.605) (-107.3767, 1.524, 21.5283) (-114.3, 1.524, 21.6027) (-121.2233, 1.524, 21.5283) (-121.2977, 1.524, 14.605) (-121.2233, 1.524, 7.6817) (-109.5375, 0, -30.4927) (-102.6142, 0, -30.4183) (-102.5398, 0, -23.495) (-102.6142, 0, -16.5717) (-109.5375, 0, -16.4973) (-116.4608, 0, -16.5717) (-116.5352, 0, -23.495) (-116.4608, 0, -30.4183) (-109.5375, 1.524, -30.4927) (-102.6142, 1.524, -30.4183) (-102.5398, 1.524, -23.495) (-102.6142, 1.524, -16.5717) (-109.5375, 1.524, -16.4973) (-116.4608, 1.524, -16.5717) (-116.5352, 1.524, -23.495) (-116.4608, 1.524, -30.4183) (-109.5375, 0, -59.0677) (-102.6142, 0, -58.9933) (-102.5398, 0, -52.07) (-102.6142, 0, -45.1467) (-109.5375, 0, -45.0723) (-116.4608, 0, -45.1467) (-116.5352, 0, -52.07) (-116.4608, 0, -58.9933) (-109.5375, 1.524, -59.0677) (-102.6142, 1.524, -58.9933) (-102.5398, 1.524, -52.07) (-102.6142, 1.524, -45.1467) (-109.5375, 1.524, -45.0723) (-116.4608, 1.524, -45.1467) (-116.5352, 1.524, -52.07) (-116.4608, 1.524, -58.9933) (-128.5875, 1.524, -59.0677) (-121.6642, 1.524, -58.9933) (-121.5898, 1.524, -52.07) (-121.6642, 1.524, -45.1467) (-128.5875, 1.524, -45.0723) (-135.5108, 1.524, -45.1467) (-135.5852, 1.524, -52.07) (-135.5108, 1.524, -58.9933) (-128.5875, 0, -59.0677) (-121.6642, 0, -58.9933) (-121.5898, 0, -52.07) (-121.6642, 0, -45.1467) (-128.5875, 0, -45.0723) (-135.5108, 0, -45.1467) (-135.5852, 0, -52.07) (-135.5108, 0, -58.9933) (-128.5875, 0, -30.4927) (-121.6642, 0, -30.4183) (-121.5898, 0, -23.495) (-121.6642, 0, -16.5717) (-128.5875, 0, -16.4973) (-135.5108, 0, -16.5717) (-135.5852, 0, -23.495) (-135.5108, 0, -30.4183) (-128.5875, 1.524, -30.4927) (-121.6642, 1.524, -30.4183) (-121.5898, 1.524, -23.495) (-121.6642, 1.524, -16.5717) (-128.5875, 1.524, -16.4973) (-135.5108, 1.524, -16.5717) (-135.5852, 1.524, -23.495) (-135.5108, 1.524, -30.4183) (-119.0625, 0, -11.4427) (-112.1392, 0, -11.3683) (-112.0648, 0, -4.445) (-112.1392, 0, 2.4783) (-119.0625, 0, 2.5527) (-125.9858, 0, 2.4783) (-126.0602, 0, -4.445) (-125.9858, 0, -11.3683) (-119.0625, 1.524, -11.4427) (-112.1392, 1.524, -11.3683) (-112.0648, 1.524, -4.445) (-112.1392, 1.524, 2.4783) (-119.0625, 1.524, 2.5527) (-125.9858, 1.524, 2.4783) (-126.0602, 1.524, -4.445) (-125.9858, 1.524, -11.3683) (-128.5875, 0, 26.6573) (-121.6642, 0, 26.7317) (-121.5898, 0, 33.655) (-121.6642, 0, 40.5783) (-128.5875, 0, 40.6527) (-135.5108, 0, 40.5783) (-135.5852, 0, 33.655) (-135.5108, 0, 26.7317) (-128.5875, 1.524, 26.6573) (-121.6642, 1.524, 26.7317) (-121.5898, 1.524, 33.655) (-121.6642, 1.524, 40.5783) (-128.5875, 1.524, 40.6527) (-135.5108, 1.524, 40.5783) (-135.5852, 1.524, 33.655) (-135.5108, 1.524, 26.7317) (-133.35, 0, 7.6073) (-126.4267, 0, 7.6817) (-126.3523, 0, 14.605) (-126.4267, 0, 21.5283) (-133.35, 0, 21.6027) (-140.2733, 0, 21.5283) (-140.3477, 0, 14.605) (-140.2733, 0, 7.6817) (-133.35, 1.524, 7.6073) (-126.4267, 1.524, 7.6817) (-126.3523, 1.524, 14.605) (-126.4267, 1.524, 21.5283) (-133.35, 1.524, 21.6027) (-140.2733, 1.524, 21.5283) (-140.3477, 1.524, 14.605) (-140.2733, 1.524, 7.6817) (-138.1125, 0, -11.4427) (-131.1892, 0, -11.3683) (-131.1148, 0, -4.445) (-131.1892, 0, 2.4783) (-138.1125, 0, 2.5527) (-145.0358, 0, 2.4783) (-145.1102, 0, -4.445) (-145.0358, 0, -11.3683) (-138.1125, 1.524, -11.4427) (-131.1892, 1.524, -11.3683) (-131.1148, 1.524, -4.445) (-131.1892, 1.524, 2.4783) (-138.1125, 1.524, 2.5527) (-145.0358, 1.524, 2.4783) (-145.1102, 1.524, -4.445) (-145.0358, 1.524, -11.3683) (-147.6375, 0, -30.4927) (-140.7142, 0, -30.4183) (-140.6398, 0, -23.495) (-140.7142, 0, -16.5717) (-147.6375, 0, -16.4973) (-154.5608, 0, -16.5717) (-154.6352, 0, -23.495) (-154.5608, 0, -30.4183) (-147.6375, 1.524, -30.4927) (-140.7142, 1.524, -30.4183) (-140.6398, 1.524, -23.495) (-140.7142, 1.524, -16.5717) (-147.6375, 1.524, -16.4973) (-154.5608, 1.524, -16.5717) (-154.6352, 1.524, -23.495) (-154.5608, 1.524, -30.4183) (-145.1281, 0, 28.2829) (-141.7025, 0, 28.3573) (-141.6281, 0, 33.9979) (-141.7025, 0, 39.6385) (-145.1281, 0, 39.7129) (-148.5537, 0, 39.6385) (-148.6281, 0, 33.9979) (-148.5537, 0, 28.3573) (-145.1281, 1.524, 28.2829) (-141.7025, 1.524, 28.3573) (-141.6281, 1.524, 33.9979) (-141.7025, 1.524, 39.6385) (-145.1281, 1.524, 39.7129) (-148.5537, 1.524, 39.6385) (-148.6281, 1.524, 33.9979) (-148.5537, 1.524, 28.3573) (-140.495, 1.524, 45.7073) (-133.5717, 1.524, 45.7817) (-133.4973, 1.524, 52.705) (-133.5717, 1.524, 59.6283) (-140.495, 1.524, 59.7027) (-147.4183, 1.524, 59.6283) (-147.4927, 1.524, 52.705) (-147.4183, 1.524, 45.7817) (-140.495, 0, 45.7073) (-133.5717, 0, 45.7817) (-133.4973, 0, 52.705) (-133.5717, 0, 59.6283) (-140.495, 0, 59.7027) (-147.4183, 0, 59.6283) (-147.4927, 0, 52.705) (-147.4183, 0, 45.7817) (-157.1625, 0, 26.6573) (-150.2392, 0, 26.7317) (-150.1648, 0, 33.655) (-150.2392, 0, 40.5783) (-157.1625, 0, 40.6527) (-164.0858, 0, 40.5783) (-164.1602, 0, 33.655) (-164.0858, 0, 26.7317) (-157.1625, 1.524, 26.6573) (-150.2392, 1.524, 26.7317) (-150.1648, 1.524, 33.655) (-150.2392, 1.524, 40.5783) (-157.1625, 1.524, 40.6527) (-164.0858, 1.524, 40.5783) (-164.1602, 1.524, 33.655) (-164.0858, 1.524, 26.7317) (-159.5425, 0, 7.6073) (-152.6192, 0, 7.6817) (-152.5448, 0, 14.605) (-152.6192, 0, 21.5283) (-159.5425, 0, 21.6027) (-166.4658, 0, 21.5283) (-166.5402, 0, 14.605) (-166.4658, 0, 7.6817) (-159.5425, 1.524, 7.6073) (-152.6192, 1.524, 7.6817) (-152.5448, 1.524, 14.605) (-152.6192, 1.524, 21.5283) (-159.5425, 1.524, 21.6027) (-166.4658, 1.524, 21.5283) (-166.5402, 1.524, 14.605) (-166.4658, 1.524, 7.6817) (-161.925, 0, -11.4427) (-155.0017, 0, -11.3683) (-154.9273, 0, -4.445) (-155.0017, 0, 2.4783) (-161.925, 0, 2.5527) (-168.8483, 0, 2.4783) (-168.9227, 0, -4.445) (-168.8483, 0, -11.3683) (-161.925, 1.524, -11.4427) (-155.0017, 1.524, -11.3683) (-154.9273, 1.524, -4.445) (-155.0017, 1.524, 2.4783) (-161.925, 1.524, 2.5527) (-168.8483, 1.524, 2.4783) (-168.9227, 1.524, -4.445) (-168.8483, 1.524, -11.3683) (-166.6875, 0, -30.4927) (-159.7642, 0, -30.4183) (-159.6898, 0, -23.495) (-159.7642, 0, -16.5717) (-166.6875, 0, -16.4973) (-173.6108, 0, -16.5717) (-173.6852, 0, -23.495) (-173.6108, 0, -30.4183) (-166.6875, 1.524, -30.4927) (-159.7642, 1.524, -30.4183) (-159.6898, 1.524, -23.495) (-159.7642, 1.524, -16.5717) (-166.6875, 1.524, -16.4973) (-173.6108, 1.524, -16.5717) (-173.6852, 1.524, -23.495) (-173.6108, 1.524, -30.4183) (-169.1969, 0, 28.2829) (-165.7713, 0, 28.3573) (-165.6969, 0, 33.9979) (-165.7713, 0, 39.6385) (-169.1969, 0, 39.7129) (-172.6225, 0, 39.6385) (-172.6969, 0, 33.9979) (-172.6225, 0, 28.3573) (-169.1969, 1.524, 28.2829) (-165.7713, 1.524, 28.3573) (-165.6969, 1.524, 33.9979) (-165.7713, 1.524, 39.6385) (-169.1969, 1.524, 39.7129) (-172.6225, 1.524, 39.6385) (-172.6969, 1.524, 33.9979) (-172.6225, 1.524, 28.3573) (-164.3075, 0, 45.7073) (-157.3842, 0, 45.7817) (-157.3098, 0, 52.705) (-157.3842, 0, 59.6283) (-164.3075, 0, 59.7027) (-171.2308, 0, 59.6283) (-171.3052, 0, 52.705) (-171.2308, 0, 45.7817) (-164.3075, 1.524, 45.7073) (-157.3842, 1.524, 45.7817) (-157.3098, 1.524, 52.705) (-157.3842, 1.524, 59.6283) (-164.3075, 1.524, 59.7027) (-171.2308, 1.524, 59.6283) (-171.3052, 1.524, 52.705) (-171.2308, 1.524, 45.7817) (-166.6875, 0, -59.0677) (-159.7642, 0, -58.9933) (-159.6898, 0, -52.07) (-159.7642, 0, -45.1467) (-166.6875, 0, -45.0723) (-173.6108, 0, -45.1467) (-173.6852, 0, -52.07) (-173.6108, 0, -58.9933) (-166.6875, 1.524, -59.0677) (-159.7642, 1.524, -58.9933) (-159.6898, 1.524, -52.07) (-159.7642, 1.524, -45.1467) (-166.6875, 1.524, -45.0723) (-173.6108, 1.524, -45.1467) (-173.6852, 1.524, -52.07) (-173.6108, 1.524, -58.9933)
sketch "スケッチ2" plane through (0, 1.524, 0) normal (0, 1, 0) x (1, 0, 0)
  line L0 (-183.1975, 68.58) -> (183.1975, 68.58)
  line L1 (183.1975, 68.58) -> (183.1975, -68.58)
  line L2 (183.1975, -68.58) -> (-183.1975, -68.58)
  line L3 (-183.1975, -68.58) -> (-183.1975, 68.58)
  line L4 (-183.1975, -68.58) -> (183.1975, 68.58) construction
  line L5 (-183.1975, 68.58) -> (183.1975, -68.58) construction
  circle A0 centre (176.8475, -62.23) radius 3
  circle A1 centre (113.1087, -52.705) radius 3.5
  circle A2 centre (4.7625, -52.705) radius 3.5
  line L6 (-26.5938, -45.6073) -> (-40.0812, -45.6073) projected
  line L7 (-26.5938, -59.7027) -> (-40.0812, -59.7027) projected
  line L8 (-33.3375, -45.6073) -> (-33.3375, -59.7027) construction
  line L9 (-116.6352, -26.9113) -> (-116.6352, -40.3987) projected
  line L10 (-121.4898, -40.3987) -> (-121.4898, -26.9113) projected
  circle A3 centre (-176.8475, 62.23) radius 3
  circle A4 centre (-96.8375, 63.5) radius 3
  circle A5 centre (-46.0375, 63.5) radius 3
  circle A6 centre (28.8925, 62.23) radius 3
  circle A7 centre (114.3, 62.23) radius 3
  circle A8 centre (114.3, 37.7825) radius 3
  circle A9 centre (113.1087, 4.445) radius 3
  circle A10 centre (84.5337, 4.445) radius 3
  line L11 (90.8863, -45.6073) -> (104.3737, -45.6073) projected
  line L12 (121.8438, -59.8027) -> (135.3312, -59.8027) projected
  line L13 (128.5875, -59.8027) -> (97.63, -45.6073) construction
  line L14 (-1.9812, -40.7527) -> (11.5062, -40.7527) construction
  line L15 (-78.1812, -40.7527) -> (-64.6938, -40.7527) construction
  circle A11 centre (-71.4375, -52.705) radius 3
  circle A12 centre (-176.8475, -62.23) radius 3
  line L16 (107.1102, 19.9182) -> (121.4898, 19.9182) construction
  line L17 (121.4898, 30.2387) -> (121.4898, 16.7513) construction
  line L18 (107.1102, 16.7513) -> (107.1102, 30.2387) construction
  line L19 (78.5352, 4.445) -> (90.5323, 4.445) construction
  line L20 (90.5323, 1.6637) -> (90.5323, -11.8237) construction
  line L21 (78.5352, -2.2987) -> (78.5352, 11.1887) construction
  line L22 (93.2688, 44.9723) -> (106.7562, 44.9723) construction
  line L23 (100.0125, 44.9723) -> (100.0125, 30.5927) construction
  line L24 (106.7562, 30.5927) -> (93.2688, 30.5927) construction
  circle A13 centre (176.8475, 37.7825) radius 3
  line L25 (173.4312, 30.5927) -> (159.9438, 30.5927) construction
  line L26 (113.1087, -52.705) -> (113.1087, 4.445) construction
  line L27 (114.3, 62.23) -> (114.3, 37.7825) construction
  line L28 (114.3, 37.7825) -> (176.8475, 37.7825) construction
  line L29 (-176.8475, -62.23) -> (176.8475, -62.23) construction
  line L30 (176.8475, -62.23) -> (176.8475, 37.7825) construction
  line L31 (114.3, 62.23) -> (28.8925, 62.23) construction
  line L32 (87.7062, 59.1677) -> (74.2188, 59.1677) construction
  line L33 (-176.8475, 62.23) -> (28.8925, 62.23) construction
  line L34 (-176.8475, 62.23) -> (-176.8475, -5.08) construction
  line L35 (-176.8475, -5.08) -> (-176.8475, -62.23) construction
  circle A14 centre (-176.8475, -5.08) radius 3
  line L36 (-155.1813, -2.6527) -> (-168.6687, -2.6527) projected
  line L37 (-161.925, -2.6527) -> (-159.5425, -7.5073) construction
  line L38 (-166.2862, -7.5073) -> (-152.7988, -7.5073) projected
  line L39 (-71.4375, -52.705) -> (4.7625, -52.705) construction
  line L40 (4.7625, -52.705) -> (113.1087, -52.705) construction
  line L41 (84.5337, 4.445) -> (113.1087, 4.445) construction
  point P0 (0, 0)
  point P1 (0, 0)
  point P2 (4.7625, -40.7527)
  point P3 (4.7625, -40.7527)
  point P4 (-71.4375, -40.7527)
  point P5 (-71.4375, -40.7527)
  point P6 (114.3, 19.9182)
  point P7 (100.0125, 37.7825)
  point P8 (-160.7337, -5.08)
  dimension "d212" = 137.16
  dimension "d213" = 366.395
  dimension "d214" = 6
  dimension "d215" = 6.35
  dimension "d216" = 6.35
  dimension "d220" = 7
  dimension "d223" = 7
  dimension "d226" = 6.35
  dimension "d227" = 6.35
  dimension "d231" = 4.8546
  dimension "d232" = 6
  dimension "d233" = 6
  dimension "d234" = 5.08
  dimension "d235" = 86.36
  dimension "d236" = 50.8
  dimension "d237" = 6
  dimension "d239" = 205.74
  dimension "d240" = 6
  dimension "d241" = 6
  dimension "d242" = 6
  dimension "d243" = 6
  dimension "d244" = 6
  dimension "d245" = 6
  dimension "d246" = 6
  dimension "d247" = 6
  dimension "d249" = 6
  constraints: 48 end point, 21 midpoint, 19 coincident, 15 centre point, 11 horizontal alignment, 8 horizontal, 8 vertical alignment, 4 point on line, 4 vertical, 3 parallel, 2 perpendicular, 1 collinear
  measures "d212" distance of L0.end L1.end
  measures "d213" distance of L1.end L2.end
  measures "d214" diameter of A0
  measures "d215" horizontal distance of L1.end L29.end
  measures "d216" horizontal distance of L1.end L29.end
  measures "d220" diameter of A1
  measures "d223" diameter of A2
  measures "d226" distance from line of L3 point (-176.848, 62.23)
  measures "d227" distance from line of L0 point (-176.848, 62.23)
  measures "d231" distance between parallel lines of L9 L10
  measures "d232" diameter of A3
  measures "d233" diameter of A4
  measures "d234" distance from line of L0 A4.centre
  measures "d235" distance from line of L3 A4.centre
  measures "d236" distance of A4.centre point (-46.038, 63.5)
  measures "d237" diameter of A5
  measures "d239" distance of L33.start point (28.892, 62.23)
  measures "d240" diameter of A6
  measures "d241" diameter of A7
  measures "d242" diameter of A8
  measures "d243" diameter of A9
  measures "d244" diameter of A10
  measures "d245" diameter of A11
  measures "d246" diameter of A12
  measures "d247" diameter of A13
  measures "d249" diameter of A14
extrude "押し出し2" add sketch "スケッチ2" against normal blind 5.0038 contours A0 | A1 | A2 | A3 | A4 | A5 | A6 | A7 | A8 | A9 | A10 | A11 | A12 | A13 | A14
